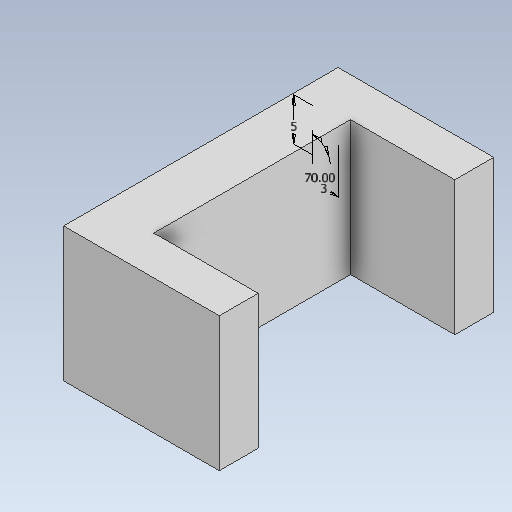
# Autodesk Inventor part: Soporte Servo SG90
Saved by Autodesk Inventor 2020.3 (Build 243373000, 373)
## iProperties
Created: 2020-11-04
Part Number: Soporte Servo SG90
Material: Generic
Document SubType Name: Modeling
Designer: juanp
Density: 1 g/cm^3
Appearance: Default
Author: juanp
Autodesk Inventor part; units mm, degrees
ref_plane "YZ Plane" through (0, 0, 0) normal (1, 0, 0) x (0, 1, 0)
ref_plane "XZ Plane" through (0, 0, 0) normal (0, 1, 0) x (-1, 0, 0)
ref_plane "XY Plane" through (0, 0, 0) normal (0, 0, 1) x (1, 0, 0)
sketch "Sketch1" plane through (0, 0, 0) normal (0, 1, 0) x (-1, 0, 0)
  line L0 (0, -11.5) -> (0, 11.5) construction
  line L1 (0, -16.05) -> (0, 16.05) construction
  line L2 (0, -16.05) -> (-12.2, -16.05)
  line L3 (-12.2, -16.05) -> (-12.2, -11.5)
  line L4 (-12.2, -11.5) -> (0, -11.5)
  line L5 (0, -11.5) -> (0, -16.05) construction
  line L6 (0, 11.5) -> (-12.2, 11.5)
  line L7 (-12.2, 11.5) -> (-12.2, 16.05)
  line L8 (-12.2, 16.05) -> (0, 16.05)
  line L9 (0, 16.05) -> (0, 11.5) construction
  line L10 (0, -16.05) -> (6, -16.05)
  line L11 (6, -16.05) -> (6, 16.05)
  line L12 (6, 16.05) -> (0, 16.05)
  line L13 (0, -11.5) -> (0, 11.5)
  point P0 (0, 0)
  point P1 (0, 0)
  dimension "d0" = 23
  dimension "d1" = 32.1
  dimension "d2" = 12.2
  dimension "d3" = 6
  constraints: 28 end point, 5 equal length, 4 perpendicular, 3 horizontal, 2 coincident, 2 midpoint, 2 vertical, 1 collinear
  measures "d0" distance of L0.start L0.end
  measures "d1" distance of L1.start L1.end
  measures "d2" distance of L1.start L2.end
  measures "d3" distance of L11.end L1.end
extrude "Extrusion1" add sketch "Sketch1" along normal blind 15.7
sketch "Sketch2" plane through (12.2, 0, -16.05) normal (0, 0, -1) x (-1, 0, 0)
  line L0 (18.2, 0) -> (18.2, 15.7) projected
  line L1 (18.2, 9.2581) -> (21.2, 10.35)
  line L2 (21.2, 10.35) -> (21.2, 5.35)
  line L3 (21.2, 5.35) -> (18.2, 6.4419)
  line L4 (18.2, 7.85) -> (21.2, 7.85) construction
  point P0 (12.2, 0)
  dimension "d6" = 3
  dimension "d7" = 70
  dimension "d8" = 5
  constraints: 8 end point, 2 midpoint, 2 point on line, 1 equal length, 1 horizontal, 1 parallel
  measures "d6" distance of L4.start L4.end
  measures "d7" angle of L2 L3
  measures "d8" distance of L1.end L2.end
body "Solid1"
